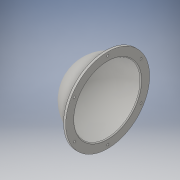
# Autodesk Inventor part: ROV Dome 4''
Saved by Autodesk Inventor 2016 (Build 200138000, 138)
## iProperties
Created: 2017-02-01
Part Number: ROV Dome 4''
Material: Generic
Document SubType Name: Modeling
Designer: Student
Density: 1 g/cm^3
Appearance: Default
Mass: 45.4784 g
Surface Area: 368.897 cm^2
Volume: 45.4784 cm^3
Author: Student
Autodesk Inventor part; units mm, degrees
ref_plane "YZ Plane" through (0, 0, 0) normal (1, 0, 0) x (0, 1, 0)
ref_plane "XZ Plane" through (0, 0, 0) normal (0, 1, 0) x (-1, 0, 0)
ref_plane "XY Plane" through (0, 0, 0) normal (0, 0, 1) x (1, 0, 0)
sketch "Sketch1" plane through (0, 0, 0) normal (0, 1, 0) x (-1, 0, 0)
  arc A0 (50.8, 0) -> (4.3366, 50.6146) centre (0, 0) ccw
  line L0 (3.175, 51.8799) -> (3.175, 60.2257)
  line L1 (0, 60.2257) -> (0, 48.8785)
  arc A1 (47.625, 0) -> (1.237, 47.6089) centre (0, 0) ccw
  line L2 (3.175, 60.2257) -> (0, 60.2257)
  line L3 (50.8, 0) -> (47.6207, 0)
  line L4 (0, 47.625) -> (0, -34.2701) construction
  line L5 (50.8, 0) -> (0, 0) construction
  arc A2 (3.175, 51.8799) -> (4.3366, 50.6146) centre (4.445, 51.8799) ccw
  arc A3 (0, 48.8785) -> (1.237, 47.6089) centre (1.27, 48.8785) ccw
  point P0 (3.175, 50.7007)
  dimension "d5" = 3.175
  dimension "d20" = 3.175
  dimension "d22" = 9.525
  dimension "d23" = 50.8
  dimension "d24" = 1.27
  constraints: 12 end point, 10 point on circle, 4 centre point, 4 point on line, 4 tangent, 2 coincident, 2 horizontal, 2 vertical, 1 equal radius, 1 perpendicular
  measures "d5" radial gap between concentric circles of A0 A1
  measures "d20" distance between parallel lines of L1 L0
  measures "d22" distance of point (3.175, 50.701) L0.end
  measures "d23" radius of A0
  measures "d24" radius of A2
revolve "Revolution1" add sketch "Sketch1" angle 360 about axis through (-50.8, 0, 0) along (1, 0, 0)
sketch "Sketch2" plane through (-3.175, 0, 0) normal (-1, 0, 0) x (0, 0, 1)
  circle A0 centre (0, 55.245) radius 1.4986
  circle A1 centre (0, 0) radius 50.7007 projected
  circle A2 centre (-47.8436, 27.6225) radius 1.4986
  circle A3 centre (-47.8436, -27.6225) radius 1.4986
  circle A4 centre (0, -55.245) radius 1.4986
  circle A5 centre (47.8436, -27.6225) radius 1.4986
  circle A6 centre (47.8436, 27.6225) radius 1.4986
  point P0 (0, 0)
  dimension "d10" = 2.9972
  dimension "d12" = 55.245
  dimension "d15" = 360
  constraints: 6 centre point, 13 other
  measures "d10" diameter of A0
  measures "d12" distance of point (0, 0) A0.centre
extrude "Extrusion1" cut sketch "Sketch2" against normal blind 254 contours A0 | A2 | A3 | A4 | A5 | A6
body "Solid1"
